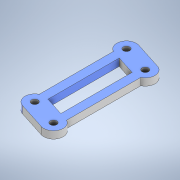
# Autodesk Inventor part: damping_system_connector
Saved by Autodesk Inventor 2021 (Build 250183000, 183)
## iProperties
Created: 2020-10-27
Part Number: damping_system_connector
Material: Generic
Document SubType Name: Modeling
Designer: Mateusz
Density: 1 g/cm^3
Appearance: Default
Author: Mateusz
Autodesk Inventor part; units mm, degrees
ref_plane "YZ Plane" through (0, 0, 0) normal (1, 0, 0) x (0, 1, 0)
ref_plane "XZ Plane" through (0, 0, 0) normal (0, 1, 0) x (-1, 0, 0)
ref_plane "XY Plane" through (0, 0, 0) normal (0, 0, 1) x (1, 0, 0)
sketch "Sketch1" plane through (0, 0, 0) normal (0, 1, 0) x (-1, 0, 0)
  circle A0 centre (0, 0) radius 11
  arc A1 (-6, 12.0934) -> (6, 12.0934) centre (0, 0) ccw
  line L0 (-6, 13.5) -> (-6, 113.5)
  line L1 (6, 113.5) -> (6, 13.5)
  line L2 (6, 12.0934) -> (6, 13.5)
  line L3 (-6, 13.5) -> (-6, 12.0934)
  arc A2 (6, 114.9066) -> (-6, 114.9066) centre (0, 127) ccw
  circle A3 centre (0, 127) radius 11
  line L4 (6, 113.5) -> (6, 114.9066)
  line L5 (-6, 113.5) -> (-6, 114.9066)
  circle A4 centre (0, 127) radius 4.5
  circle A5 centre (0, 0) radius 4.5
  dimension "d0" = 22
  dimension "d4" = 100
  dimension "d7" = 9
  dimension "d8" = 9
  constraints: 12 end point, 6 centre point, 5 coincident, 4 point on circle, 2 point on line, 1 collinear, 1 parallel, 1 vertical
  measures "d0" diameter of A0
  measures "d4" distance of L0.start L0.end
  measures "d7" diameter of A4
  measures "d8" diameter of A5
extrude "Extrusion1" add sketch "Sketch1" against normal blind 3 contours A0 | L3 L0 L5 A2 L4 L1 L2 A1 | A3
extrude "Extrusion2" add sketch "Sketch1" along normal blind 6 contours A0 | L3 L0 L5 A2 L4 L1 L2 A1 | A3
sketch "Sketch2" plane through (0, -3, 0) normal (0, -1, 0) x (1, 0, 0)
  arc A0 (-6, 12.0934) -> (6, 12.0934) centre (0, 0) ccw projected
  line L0 (6, 12.0934) -> (6, 114.9066) projected
  arc A1 (6, 114.9066) -> (-6, 114.9066) centre (0, 127) ccw projected
  line L1 (-6, 114.9066) -> (-6, 12.0934) projected
  circle A2 centre (0, 0) radius 4.5 projected
  circle A3 centre (0, 127) radius 4.5 projected
extrude "Extrusion3" add sketch "Sketch2" along normal blind 1
sketch "Sketch4" plane through (0, 6, 0) normal (0, 1, 0) x (1, 0, 0)
  line L0 (-6, -12.0934) -> (-6, -114.9066) projected
  line L1 (-6, -63.5) -> (6, -63.5)
  line L2 (6, -114.9066) -> (6, -12.0934) projected
  circle A0 centre (0, -63.5) radius 1.45
  point P0 (0, 0)
  dimension "d17" = 2.9
  constraints: 3 midpoint, 2 end point, 1 centre point
  measures "d17" diameter of A0
extrude "Extrusion5" cut sketch "Sketch4" against normal up to surface (10 mm away)
sketch "Sketch5" plane through (0, 6, 0) normal (0, 1, 0) x (1, 0, 0)
  arc A0 (6, -12.0934) -> (-6, -12.0934) centre (0, 0) ccw projected
  arc A1 (44.1065, -24.2547) -> (42.2109, 0.6996) centre (38.1065, -12.1613) ccw
  arc A2 (34.002, -152.0223) -> (44.1065, -127.0679) centre (38.1065, -139.1613) ccw
  circle A3 centre (38.1065, -139.1613) radius 4.5
  circle A4 centre (38.1065, -12.1613) radius 4.5
  arc A5 (-6, -114.9066) -> (6, -114.9066) centre (0, -127) ccw projected
  line L0 (44.1065, -105.6324) -> (44.1065, -127.0679)
  line L1 (32.1065, -105.6324) -> (32.1065, -123.0757)
  line L2 (44.1065, -105.6324) -> (44.1065, -24.2547)
  line L3 (32.1065, -105.6324) -> (32.1065, -24.2547)
  line L4 (-4.1044, -139.8609) -> (35.9659, -152.649)
  line L5 (6, -114.744) -> (32.1065, -123.0757)
  line L6 (6, -114.9066) -> (6, -12.0934) projected
  line L7 (6, -16.0857) -> (34.002, -25.0223)
  line L8 (4.1044, 12.8609) -> (42.2109, 0.6996)
  point P0 (32.1065, -24.4173)
  constraints: 16 end point, 8 tangent, 7 point on circle, 5 point on line, 4 centre point, 2 coincident, 2 vertical, 1 parallel, 2 other
extrude "Extrusion6" add sketch "Sketch5" against normal up to surface (10 mm away) contours A0 L8 A1 L2 L0 A2 L4 A5 L6 L5 L1 L3 L7
sketch "Sketch6" plane through (0, 6, 0) normal (0, 1, 0) x (1, 0, 0)
  circle A0 centre (0, -63.5) radius 1.45 projected
  point P0 (0, 0)
extrude "Extrusion7" add sketch "Sketch6" against normal up to surface (10 mm away)
body "Solid1"
